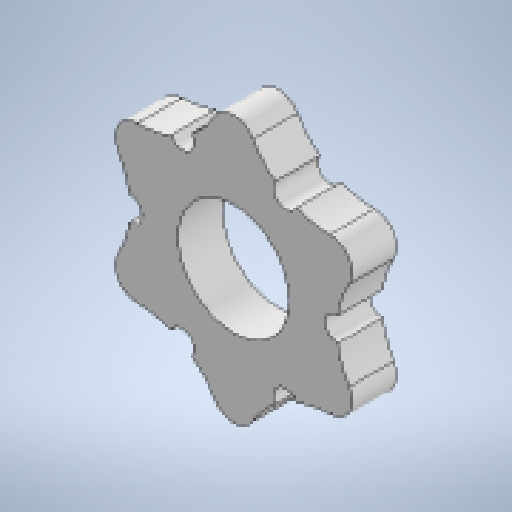
# Autodesk Inventor part: Gyro Core
Saved by Autodesk Inventor 2023.2 (Build 272271000, 271)
## iProperties
Created: 2023-06-11
Part Number: Gyro Core
Material: UHMW, White
Document SubType Name: Modeling
Designer: Nathan Cai
Density: 0.94 g/cm^3
Appearance: Smooth - White
Author: Nathan Cai
Autodesk Inventor part; units mm, degrees
ref_plane "YZ Plane" through (0, 0, 0) normal (1, 0, 0) x (0, 1, 0)
ref_plane "XZ Plane" through (0, 0, 0) normal (0, 1, 0) x (-1, 0, 0)
ref_plane "XY Plane" through (0, 0, 0) normal (0, 0, 1) x (1, 0, 0)
sketch "Sketch1" plane through (0, 0, 0) normal (0, 0, 1) x (1, 0, 0)
  circle A0 centre (0, 0) radius 7.9375
  circle A1 centre (0, 0) radius 19.05 construction
  line L0 (0, 0) -> (0, 19.05) construction
  circle A2 centre (0, 15.875) radius 3.175
  circle A3 centre (-13.7482, 7.9375) radius 3.175
  circle A4 centre (-13.7482, -7.9375) radius 3.175
  circle A5 centre (0, -15.875) radius 3.175
  circle A6 centre (13.7482, -7.9375) radius 3.175
  circle A7 centre (13.7482, 7.9375) radius 3.175
  arc A8 (-13.7482, 11.1125) -> (-2.7496, 17.4625) centre (-13.7482, 23.8125) ccw
  circle A9 centre (-7.3982, 12.814) radius 1.7526
  circle A10 centre (-14.7963, 0) radius 1.7526
  arc A11 (-16.4978, -6.35) -> (-16.4978, 6.35) centre (-27.4963, 0) ccw
  circle A12 centre (-7.3982, -12.814) radius 1.7526
  arc A13 (-2.7496, -17.4625) -> (-13.7482, -11.1125) centre (-13.7482, -23.8125) ccw
  circle A14 centre (7.3982, -12.814) radius 1.7526
  arc A15 (13.7482, -11.1125) -> (2.7496, -17.4625) centre (13.7482, -23.8125) ccw
  circle A16 centre (14.7963, 0) radius 1.7526
  arc A17 (16.4978, 6.35) -> (16.4978, -6.35) centre (27.4963, 0) ccw
  circle A18 centre (7.3982, 12.814) radius 1.7526
  arc A19 (2.7496, 17.4625) -> (13.7482, 11.1125) centre (13.7482, 23.8125) ccw
  point P0 (-16.4978, 6.35)
  point P1 (-14.9172, 1.7484)
  point P2 (-14.9172, -1.7484)
  point P3 (-13.7482, -11.1125)
  point P4 (-8.9728, -12.0445)
  point P5 (-5.9444, -13.7929)
  point P6 (-2.7496, -17.4625)
  point P7 (2.7496, -17.4625)
  point P8 (5.9444, -13.7929)
  point P9 (8.9728, -12.0445)
  point P10 (13.7482, -11.1125)
  point P11 (16.4978, -6.35)
  point P12 (14.9172, -1.7484)
  point P13 (14.9172, 1.7484)
  point P14 (16.4978, 6.35)
  point P15 (8.9728, 12.0445)
  point P16 (5.9444, 13.7929)
  point P17 (2.7496, 17.4625)
  point P18 (-5.9444, 13.7929)
  point P19 (-8.9728, 12.0445)
  dimension "d1" = 38.1
  dimension "d2" = 6.35
  dimension "d0" = 15.875
  dimension "d5" = 360
  dimension "d7" = 12.7
  dimension "d8" = 3.5052
  dimension "d11" = 360
  constraints: 17 centre point, 13 point on circle, 2 coincident, 2 end point, 1 point on line, 1 vertical, 1 vertical alignment, 60 other
  measures "d0" diameter of A0
  measures "d7" radius of A8
  measures "d8" diameter of A9
extrude "Extrusion1" add sketch "Sketch1" along normal blind 6.35 contours A2 | A2 A19 A18 A7 A17 A16 A6 A15 A14 A5 A13 A12 A4 A11 A10 A3 A8 A9 | A7 | A3 | A6 | A4 | A5
body "Solid1"
